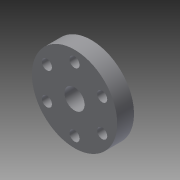
# Autodesk Inventor part: hub_6mm_M3
Saved by Autodesk Inventor 2015 (Build 190159000, 159)
## iProperties
Created: 2015-06-21
Part Number: hub_6mm_M3
Material: Générique
Document SubType Name: Modeling
Designer: astralien3000
Density: 1 g/cm^3
Appearance: Par défaut
d0: 25,400 mm
d1: 5,000 mm
d2: 0,00 deg
d3: 12,000 mm
d4: 4,200 mm
d5: 0,00 deg
d6: 6,000 mm
d8: 0,00 deg
d9: 3,000 mm
d10: 9,500 mm
d11: 0,000 mm
d12: 6,000 nd
d17: 0,00 deg
d14: 360,00 deg
Author: astralien3000
Autodesk Inventor part; units mm, degrees
ref_plane "YZ Plane" through (0, 0, 0) normal (1, 0, 0) x (0, 1, 0)
ref_plane "XZ Plane" through (0, 0, 0) normal (0, 1, 0) x (-1, 0, 0)
ref_plane "XY Plane" through (0, 0, 0) normal (0, 0, 1) x (1, 0, 0)
sketch "Esquisse1" plane through (0, 0, 0) normal (0, 1, 0) x (-1, 0, 0)
  circle A0 centre (0, 0) radius 12.7
  dimension "d0" = 25.4
  constraints: 1 centre point, 1 coincident
  measures "d0" diameter of A0
extrude "Extrusion1" add sketch "Esquisse1" along normal blind 5
sketch "Esquisse2" plane through (0, 5, 0) normal (0, 1, 0) x (1, 0, 0)
  circle A0 centre (0, 0) radius 12.7 projected
  circle A1 centre (0, 0) radius 6
  dimension "d3" = 12
  constraints: 1 centre point, 1 coincident
  measures "d3" diameter of A1
extrude "Extrusion2" add sketch "Esquisse2" along normal blind 4.2 contours A1
sketch "Esquisse3" plane through (0, 9.2, 0) normal (0, 1, 0) x (1, 0, 0)
  circle A0 centre (0, 0) radius 6 projected
  circle A1 centre (0, 0) radius 3
  dimension "d6" = 6
  constraints: 1 centre point, 1 coincident
  measures "d6" diameter of A1
extrude "Extrusion3" cut sketch "Esquisse3" against normal through all contours A1
sketch "Esquisse4" plane through (0, 0, 0) normal (0, -1, 0) x (1, 0, 0)
  circle A0 centre (0, 0) radius 3 projected
  circle A1 centre (0, 9.5) radius 1.5
  circle A2 centre (-8.2272, 4.75) radius 1.5
  circle A3 centre (-8.2272, -4.75) radius 1.5
  circle A4 centre (0, -9.5) radius 1.5
  circle A5 centre (8.2272, -4.75) radius 1.5
  circle A6 centre (8.2272, 4.75) radius 1.5
  dimension "d9" = 3
  dimension "d10" = 9.5
  dimension "d11" = 0
  dimension "d14" = 360
  constraints: 6 centre point, 13 other
  measures "d9" diameter of A1
  measures "d10" distance of A0.centre A1.centre
  measures "d11" horizontal distance of A0.centre A1.centre
extrude "Extrusion4" cut sketch "Esquisse4" against normal through all contours A1 | A2 | A3 | A4 | A5 | A6
